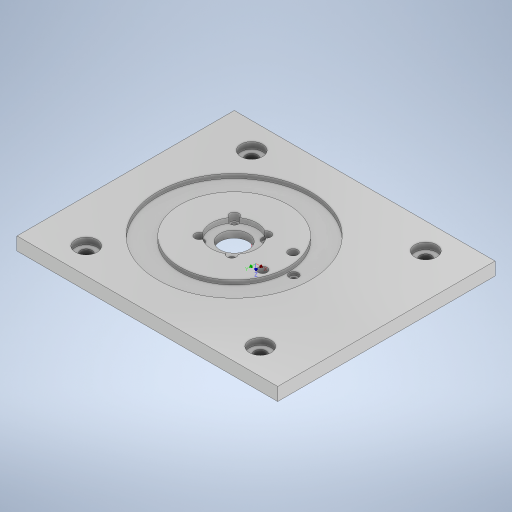
# Autodesk Inventor part: axis_1_top_frame
Saved by Autodesk Inventor 2024.2 (Build 282272000, 272)
## iProperties
Created: 2023-08-26
Part Number: axis_1_top_frame
Material: Aluminum 6061-AHC
Document SubType Name: Modeling
Designer: chanh
Density: 2.7 g/cm^3
Appearance: Aluminum - Dark
Author: chanh
Autodesk Inventor part; units mm, degrees
ref_plane "YZ Plane" through (0, 0, 0) normal (1, 0, 0) x (0, 1, 0)
ref_plane "XZ Plane" through (0, 0, 0) normal (0, 1, 0) x (-1, 0, 0)
ref_plane "XY Plane" through (0, 0, 0) normal (0, 0, 1) x (1, 0, 0)
sketch "Sketch1" plane through (0, 0, 0) normal (0, 1, 0) x (-1, 0, 0)
  line L0 (60, 50) -> (-60, 50)
  line L1 (-60, 50) -> (-60, -50)
  line L2 (-60, -50) -> (60, -50)
  line L3 (60, -50) -> (60, 50)
  line L4 (60, 50) -> (-60, -50) construction
  line L5 (-60, 50) -> (60, -50) construction
  point P0 (0, 0)
  dimension "d0" = 120
  dimension "d1" = 100
  constraints: 12 end point, 2 midpoint, 2 parallel, 1 horizontal, 1 perpendicular
  measures "d0" distance of L2.end L1.end
  measures "d1" distance of L1.end L0.end
extrude "Extrusion1" add sketch "Sketch1" along normal blind 6
sketch "Sketch5" plane through (0, 6, 0) normal (0, 1, 0) x (1, 0, 0)
  circle A0 centre (-10.05, 0) radius 1.2295 projected
  circle A1 centre (-10.05, 0) radius 10.4
  point P0 (0, 0)
  dimension "d16" = 20.8
  constraints: 1 centre point, 1 coincident
  measures "d16" diameter of A1
extrude "Extrusion3" cut sketch "Sketch5" against normal blind 2.3 contours A0 | A1
hole "Hole1" at (-18.05, 6, -8.07) at (-18.05, 6, 8.07) at (-3.15, 6, 8) at (-3.15, 6, -8) at (10.07, 6, 7) at (17.37, 6, 0) at (10.07, 6, -7) direction (0, -1, 0) diameter 2.1 end through all
sketch "Sketch8" plane through (0, 6, 0) normal (0, 1, 0) x (1, 0, 0)
  arc A0 (-17.650182, -7.0991) -> (-17.08262, -7.661739) centre (-18.05, -8.07) ccw
  arc A1 (-17.08262, 7.661739) -> (-17.650182, 7.0991) centre (-18.05, 8.07) ccw
  arc A2 (-4.068914, -8.508032) -> (-2.512532, -7.165653) centre (-3.15, -8) ccw
  arc A3 (-2.512532, 7.165653) -> (-4.068914, 8.508032) centre (-3.15, 8) ccw
  circle A4 centre (10.07, -7) radius 1.05
  circle A5 centre (17.37, 0) radius 1.05
  circle A6 centre (10.07, 7) radius 1.05
  circle A7 centre (-18.05, -8.07) radius 2.05
  circle A8 centre (-18.05, 8.07) radius 2.05
  circle A9 centre (-3.15, -8) radius 2.05
  circle A10 centre (-3.15, 8) radius 2.05
  circle A11 centre (10.07, 7) radius 2.05
  circle A12 centre (10.07, -7) radius 2.05
  circle A13 centre (17.37, 0) radius 2.05
  point P0 (0, 0)
  dimension "d31" = 4.1
  constraints: 7 centre point, 7 coincident, 6 equal radius
  measures "d31" diameter of A7
extrude "Extrusion6" cut sketch "Sketch8" against normal blind 3.5 contours A4 | A5 | A6 | A7 | A8 | A9 | A10 | A11 | A12 | A13
sketch "Sketch11" plane through (0, 6, 0) normal (0, 1, 0) x (1, 0, 0)
  circle A0 centre (-10.05, 0) radius 25 projected
  circle A1 centre (-10.05, 0) radius 35 projected
  circle A2 centre (-10.05, 0) radius 24.85
  circle A3 centre (-10.05, 0) radius 35.15
  point P0 (0, 0)
  dimension "d38" = 0.15
  dimension "d39" = 0.15
  constraints: 2 centre point
  measures "d38" radial gap between concentric circles of A0 A2
  measures "d39" radial gap between concentric circles of A1 A3
sketch "Sketch11 outline for Extrusion9" plane through (0, 6, 0) normal (0, 1, 0) x (1, 0, 0)
  circle A0 centre (-10.05, 0) radius 35.15
  circle A1 centre (-10.05, 0) radius 24.85
extrude "Extrusion9" cut sketch "Sketch11 outline for Extrusion9" against normal blind 2
sketch "Sketch12" plane through (0, 6, 0) normal (0, 1, 0) x (1, 0, 0)
  line L0 (-44.2, 50.07) -> (-44.2, -50.07) construction
  line L1 (-35.9, 50.07) -> (-35.9, -50.07) construction
  line L2 (35.9, 50.07) -> (35.9, -50.07) construction
  line L3 (44.2, 50.07) -> (44.2, -50.07) construction
  line L4 (60, 50) -> (-60, 50) projected
  line L5 (-40.05, -50.07) -> (-40.05, 50) construction
  line L6 (40.05, -50.07) -> (40.05, 50) construction
  line L7 (-44.2, -50.07) -> (-35.9, -50.07) construction
  line L8 (35.9, -50.07) -> (44.2, -50.07) construction
  line L9 (-60, 50) -> (-60, -50) projected
  line L10 (60, -50) -> (60, 50) projected
  line L11 (-60, 0) -> (60, 0) construction
  point P0 (0, 0)
  point P1 (-40.05, -38.07)
  point P2 (40.05, -38.07)
  point P3 (-40.05, 38.07)
  point P4 (40.05, 38.07)
  dimension "d42" = 12
  constraints: 10 end point, 4 midpoint, 4 point on line, 2 symmetric about line, 2 vertical, 1 horizontal, 1 horizontal alignment
  measures "d42" distance from line of point (-40.05, -38.07) L7
hole "Hole2" at (-40.05, 6, 38.07) at (40.05, 6, 38.07) at (-40.05, 6, -38.07) at (40.05, 6, -38.07) direction (0, -1, 0) diameter 5.2 end through all counterbore diameter 10 counterbore depth 3
sketch "Sketch13" plane through (0, 0, 0) normal (0, -1, 0) x (1, 0, 0)
  circle A0 centre (-10.05, 0) radius 24.85 projected
  line L0 (-19.05, 10.07) -> (19.05, 10.07)
  line L1 (20.05, 9.07) -> (20.05, -9.07)
  line L2 (19.05, -10.07) -> (-19.05, -10.07)
  line L3 (-20.05, -9.07) -> (-20.05, 9.07)
  arc A1 (-19.05, 10.07) -> (-20.05, 9.07) centre (-19.05, 9.07) ccw
  arc A2 (20.05, 9.07) -> (19.05, 10.07) centre (19.05, 9.07) ccw
  arc A3 (19.05, -10.07) -> (20.05, -9.07) centre (19.05, -9.07) ccw
  arc A4 (-20.05, -9.07) -> (-19.05, -10.07) centre (-19.05, -9.07) ccw
  point P0 (0, 0)
  point P1 (20.05, -10.07)
  point P2 (20.05, 10.07)
  point P3 (-20.05, -10.07)
  point P4 (-20.05, 0)
  dimension "d50" = 40.1
  dimension "d51" = 20.14
  dimension "d52" = 10
  dimension "d53" = 1
  constraints: 8 end point, 8 point on circle, 8 tangent, 6 point on line, 4 centre point, 3 equal radius, 2 parallel, 1 horizontal, 1 horizontal alignment, 1 midpoint, 1 perpendicular
  measures "d50" distance of point (20.05, -10.07) point (-20.05, -10.07)
  measures "d51" distance of point (20.05, 10.07) point (20.05, -10.07)
  measures "d52" distance of point (-20.05, 0) A0.centre
  measures "d53" radius of A1
extrude "Extrusion10" cut sketch "Sketch13" against normal blind 0.5 contours A0 L2 A4 L3 A1 L0 | A0 L0 A2 L1 A3 L2 picked at (-7.766667, 0)
sketch "Sketch14" plane through (0, 0.5, 0) normal (0, -1, 0) x (1, 0, 0)
  circle A0 centre (-10.05, 0) radius 24.85 projected
  circle A1 centre (-10.05, 0) radius 6.5
  point P0 (0, 0)
  dimension "d56" = 13
  constraints: 1 centre point, 1 coincident
  measures "d56" diameter of A1
extrude "Extrusion11" cut sketch "Sketch14" against normal through all contours A1
body "Solid1"
